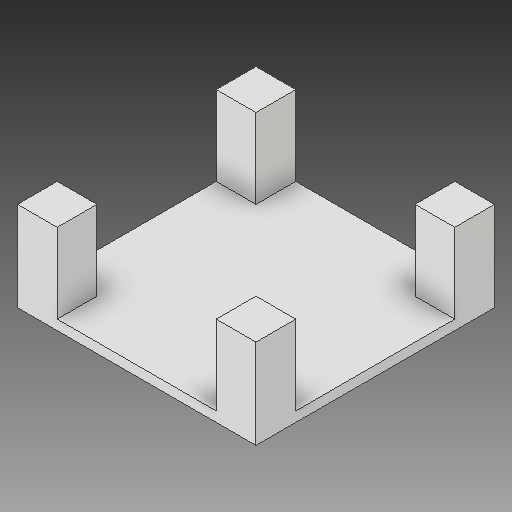
# Autodesk Inventor part: FalseFloor
Saved by Autodesk Inventor 2017 (Build 210142000, 142)
## iProperties
Created: 2017-02-25
Part Number: FalseFloor
Material: ABS Plastic
Document SubType Name: Modeling
Designer: aribu
Density: 1.06 g/cm^3
Appearance: Smooth - White
Mass: 144.16 g
Surface Area: 440 cm^2
Volume: 136 cm^3
Author: aribu
Autodesk Inventor part; units mm, degrees
ref_plane "YZ Plane" through (0, 0, 0) normal (1, 0, 0) x (0, 1, 0)
ref_plane "XZ Plane" through (0, 0, 0) normal (0, 1, 0) x (-1, 0, 0)
ref_plane "XY Plane" through (0, 0, 0) normal (0, 0, 1) x (1, 0, 0)
sketch "Sketch1" plane through (0, 0, 0) normal (0, 1, 0) x (-1, 0, 0)
  line L0 (60, -60) -> (-60, -60)
  line L1 (-60, -60) -> (-60, 60)
  line L2 (-60, 60) -> (60, 60)
  line L3 (60, 60) -> (60, -60)
  point P0 (0, 0)
  dimension "d0" = 120
  dimension "d1" = 120
  dimension "d2" = 60
  dimension "d3" = 60
  constraints: 8 end point, 2 parallel, 1 horizontal, 1 perpendicular
  measures "d0" distance of L0.start L0.end
  measures "d1" distance of L0.end L1.end
  measures "d2" distance from line of L0 point (0, 0)
  measures "d3" distance from line of L1 point (0, 0)
extrude "Extrusion1" add sketch "Sketch1" along normal blind 5
sketch "Sketch2" plane through (0, 5, 0) normal (0, 1, 0) x (1, 0, 0)
  line L0 (-40, 40) -> (-60, 40)
  line L1 (-60, 40) -> (-60, 60)
  line L2 (-60, 60) -> (-40, 60)
  line L3 (-40, 60) -> (-40, 40)
  line L4 (60, -60) -> (40, -60)
  line L5 (40, -60) -> (40, -40)
  line L6 (40, -40) -> (60, -40)
  line L7 (60, -40) -> (60, -60)
  line L8 (60, 60) -> (60, -60) projected
  line L9 (-60, -60) -> (60, -60) projected
  line L10 (60, 60) -> (-60, 60) projected
  line L11 (60, 60) -> (40, 60)
  line L12 (40, 60) -> (40, 40)
  line L13 (40, 40) -> (60, 40)
  line L14 (60, 40) -> (60, 60)
  line L15 (-60, 60) -> (-60, -60) projected
  line L16 (-60, -60) -> (-40, -60)
  line L17 (-40, -60) -> (-40, -40)
  line L18 (-40, -40) -> (-60, -40)
  line L19 (-60, -40) -> (-60, -60)
  point P0 (0, 0)
  dimension "d6" = 20
  dimension "d7" = 20
  dimension "d8" = 20
  dimension "d9" = 20
  dimension "d10" = 0
  dimension "d11" = 0
  dimension "d12" = 20
  dimension "d13" = 20
  dimension "d14" = 20
  dimension "d15" = 20
  constraints: 32 end point, 8 parallel, 4 horizontal, 4 perpendicular
  measures "d6" distance of L2.end L0.start
  measures "d7" distance of L0.start L0.end
  measures "d8" distance of L6.end L4.start
  measures "d9" distance of L4.start L4.end
  measures "d10" distance between parallel lines of L8 L7
  measures "d11" distance between parallel lines of L9 L4
  measures "d12" distance of L17.end L18.end
  measures "d13" distance of L16.end L17.end
  measures "d14" distance of L11.end L12.end
  measures "d15" distance of L12.end L13.end
extrude "Extrusion2" add sketch "Sketch2" along normal blind 40 contours L0 L1 L2 L3 | L18 L17 L9 L15 | L10 L8 L13 L12 | L5 L6 L7 L4
equation "\"d1\" = d0"
equation "\"d2\" = 0.5 * d0"
equation "\"d3\" = 0.5 * d0"
equation "\"d7\" = d6"
equation "\"d8\" = d6"
equation "\"d9\" = d6"
equation "\"d12\" = d6"
equation "\"d13\" = d6"
equation "\"d14\" = d6"
equation "\"d15\" = d6"
body "Solid1"
